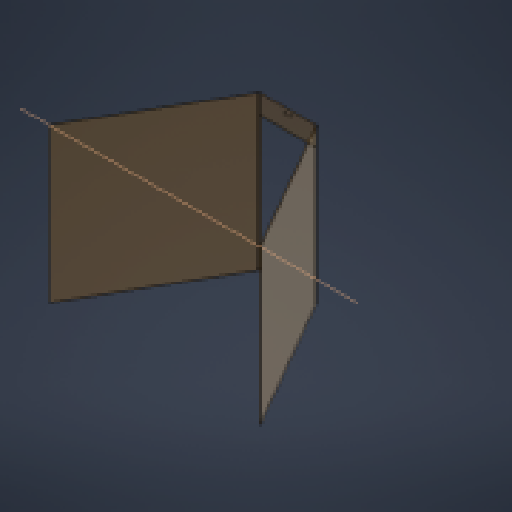
# Autodesk Inventor part: hopper
Saved by Autodesk Inventor 2024.3 (Build 283343000, 343)
## iProperties
Created: 2025-03-05
Part Number: hopper
Material: Polycarbonate, Smoke
Document SubType Name: Sheet Metal
Designer: Marcus Tannini
Density: 1.2 g/cm^3
Sheet Metal Rule: Default
Appearance: Polycarbonate - Smoked
Mass: 1340.69 g
Surface Area: 7457.91 cm^2
Volume: 1117.24 cm^3
Author: Marcus Tannini
Autodesk Inventor part; units mm, degrees
ref_plane "YZ Plane" through (0, 0, 0) normal (1, 0, 0) x (0, 1, 0)
ref_plane "XZ Plane" through (0, 0, 0) normal (0, 1, 0) x (-1, 0, 0)
ref_plane "XY Plane" through (0, 0, 0) normal (0, 0, 1) x (1, 0, 0)
sketch "Sketch1" plane through (0, 0, 0) normal (0, 0, 1) x (1, 0, 0)
  line L0 (-76.2, -203.2) -> (76.2, -203.2)
  line L1 (76.2, -203.2) -> (76.2, 203.2)
  line L2 (76.2, 203.2) -> (-76.2, 203.2)
  line L3 (-76.2, 203.2) -> (-76.2, -203.2)
  line L4 (-76.2, -203.2) -> (76.2, 203.2) construction
  line L5 (76.2, -203.2) -> (-76.2, 203.2) construction
  point P0 (0, 0)
  dimension "d0" = 152.4
  dimension "d1" = 406.4
  measures "d0" distance of L2.end L1.end
  measures "d1" distance of L0.end L1.end
extrude "Plate1" add sketch "Sketch1" along normal blind 3.048
sketch "Sketch2" plane through (73.7032, 203.2, 1.7483) normal (0.819152, 0, -0.5735764) x (0, 1, 0)
  line L0 (-406.4, 0) -> (0, 0)
  line L1 (0, 0) -> (0, 508)
  line L2 (0, 508) -> (-406.4, 508)
  line L3 (-406.4, 508) -> (-406.4, 0)
  constraints: 6 end point, 1 horizontal, 1 perpendicular, 1 vertical
edge flange "Flange1" height 508 angle 55 thickness 3.048 bend radius 3.048 thickness toward (0.819152, 0, -0.5735764) relief tear relief width 3.048 relief depth 1.524 corner gap 3.048 corner form 0 edges at (76.2, 0, 3.048) (-76.2, 0, 3.048) wall of the first edge with corners at (73.7032, -203.2, 1.7483) (73.7032, 203.2, 1.7483) (365.0801, 203.2, 417.8775) (365.0801, -203.2, 417.8775)
bend "Bend1"
corner "Corner1"
sketch "Sketch3" plane through (0, 0, 3.048) normal (0, 0, 1) x (1, 0, 0)
  line L0 (-78.0202, -203.2) -> (-78.0202, 152.4)
  line L1 (-78.0202, 152.4) -> (78.0202, 152.4)
  line L2 (78.0202, 152.4) -> (78.0202, -203.2)
  line L3 (-158.75, -203.2) -> (-78.0202, 152.4)
  line L4 (158.75, -203.2) -> (78.0202, 152.4)
  line L5 (-75.5234, -203.2) -> (-365.0801, -203.2) projected
  line L6 (75.5234, -203.2) -> (365.0801, -203.2) projected
  line L7 (-158.75, -203.2) -> (158.75, -203.2)
  line L8 (-78.0202, 203.2) -> (-78.0202, -203.2) construction
  line L9 (78.0202, -203.2) -> (78.0202, 203.2) projected
  line L10 (-73.0266, 203.2) -> (73.0266, 203.2) projected
  line L11 (73.0266, -203.2) -> (-73.0266, -203.2) projected
  point P0 (0, -203.2)
  point P1 (0, -203.2)
  dimension "d25" = 317.5
  dimension "d28" = 50.8
  constraints: 12 end point, 3 collinear, 3 point on line, 2 midpoint, 1 coincident, 1 horizontal, 1 parallel
  measures "d25" distance of L3.start L4.start
  measures "d28" distance between parallel lines of L10 L1
extrude "Cut1" cut sketch "Sketch3" against normal mid plane 508
sketch "Sketch4" plane through (0, 0, 3.048) normal (0, 0, 1) x (1, 0, 0)
  line L0 (-73.0266, 152.4) -> (73.0266, 152.4) construction
  line L1 (73.0266, 152.4) -> (73.0266, 203.2) construction
  line L2 (-73.0266, 203.2) -> (73.0266, 203.2) construction
  line L3 (-73.0266, 203.2) -> (-73.0266, 152.4) construction
  line L4 (0, 203.2) -> (0, 152.4) construction
  line L5 (0, 190.5) -> (6.35, 190.5)
  point P0 (0, 0)
  point P1 (-6.35, 190.5)
  dimension "d16" = 6.35
  dimension "d17" = 12.7
  constraints: 4 end point, 2 midpoint, 1 coincident, 1 horizontal, 1 point on line, 1 symmetric about line
  measures "d16" distance of L5.start L5.end
  measures "d17" distance between parallel lines of L2 L5
hole "Hole1" at (6.35, 190.5, 3.048) at (-6.35, 190.5, 3.048) direction (0, 0, -1) diameter 5.1054 end through all clearance for "Flat Head Machine Screw (82)" size "#10" standard "Ansi Unified Screw Threads"
equation "\"d23\" = Thickness"
equation "\"d2\" = Thickness"
equation "\"d3\" = BendReliefWidth"
equation "\"d4\" = BendReliefDepth"
equation "\"d5\" = MinimumRemnant"
equation "\"d6\" = TransitionRadius"
equation "\"d9\" = BendRadius"
equation "\"d10\" = CornerReliefSize"
equation "\"d11\" = GapSize"
equation "\"d12\" = JacobiRadiusSize"
equation "\"BendRadius\" = Thickness"
equation "\"BendReliefWidth\" = Thickness"
equation "\"BendReliefDepth\" = 0.5 * Thickness"
equation "\"CornerReliefSize\" = 4 * Thickness"
equation "\"MinimumRemnant\" = 2 * Thickness"
equation "\"TransitionRadius\" = BendRadius"
equation "\"JacobiRadiusSize\" = BendRadius"
equation "\"GapSize\" = Thickness"
equation "\"Thickness\" = 3.048"
body "Solid1"
